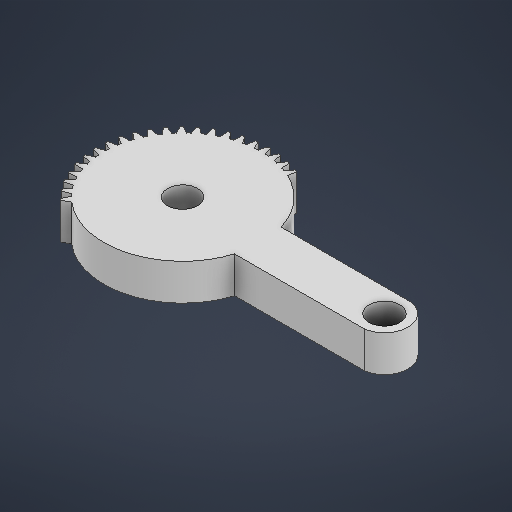
# Autodesk Inventor part: innerGear
Saved by Autodesk Inventor 2026.2 (Build 302298000, 298)
## iProperties
Created: 2026-04-07
Part Number: innerGear
Material: Generic
Document SubType Name: Modeling
Designer: Brian Wang
Density: 1 g/cm^3
Appearance: Default
Author: Brian Wang
Autodesk Inventor part; units mm, degrees
ref_plane "YZ Plane" through (0, 0, 0) normal (1, 0, 0) x (0, 1, 0)
ref_plane "XZ Plane" through (0, 0, 0) normal (0, 1, 0) x (-1, 0, 0)
ref_plane "XY Plane" through (0, 0, 0) normal (0, 0, 1) x (1, 0, 0)
sketch "Sketch1" plane through (0, 0, 0) normal (0, 1, 0) x (-1, 0, 0)
  circle A0 centre (0, 0) radius 11
  line L0 (0, 0) -> (21.5969, 0.9429) construction
  line L1 (0, 0) -> (22.384, -0.9773) construction
  line L2 (0, 0) -> (25.2479, 0) construction
  line L3 (10.9895, 0.4798) -> (12.0415, 0.1582)
  line L4 (10.9895, 0.4798) -> (12.0895, 0.4798) construction
  line L5 (10.9895, -0.4798) -> (12.0415, -0.1582)
  line L6 (12.0415, -0.1582) -> (12.0415, 0.1582)
  line L7 (10.9561, 0.9815) -> (11.9561, 1.4397)
  line L8 (11.9561, 1.4397) -> (11.9142, 1.7533)
  line L9 (10.8289, 1.9326) -> (11.9142, 1.7533)
  line L10 (10.7293, 2.4254) -> (11.6597, 3.0122)
  line L11 (11.6597, 3.0122) -> (11.5765, 3.3175)
  line L12 (10.4771, 3.3513) -> (11.5765, 3.3175)
  line L13 (10.313, 3.8266) -> (11.1574, 4.5315)
  line L14 (11.1574, 4.5315) -> (11.0345, 4.8231)
  line L15 (9.9402, 4.7109) -> (11.0345, 4.8231)
  line L16 (9.7146, 5.1602) -> (10.4581, 5.9708)
  line L17 (10.4581, 5.9708) -> (10.2976, 6.2435)
  line L18 (9.2279, 5.9872) -> (10.2976, 6.2435)
  line L19 (8.9446, 6.4026) -> (9.5741, 7.3047)
  line L20 (9.5741, 7.3047) -> (9.3789, 7.5537)
  line L21 (8.3526, 7.1578) -> (9.3789, 7.5537)
  line L22 (8.0168, 7.532) -> (8.521, 8.5096)
  line L23 (8.521, 8.5096) -> (8.2945, 8.7306)
  line L24 (7.3298, 8.2021) -> (8.2945, 8.7306)
  line L25 (6.9474, 8.5284) -> (7.3176, 9.5643)
  line L26 (7.3176, 9.5643) -> (7.0638, 9.7532)
  line L27 (6.1776, 9.1015) -> (7.0638, 9.7532)
  line L28 (5.7553, 9.3743) -> (5.9849, 10.45)
  line L29 (5.9849, 10.45) -> (5.7083, 10.6037)
  line L30 (4.9164, 9.8402) -> (5.7083, 10.6037)
  line L31 (4.4616, 10.0546) -> (4.5465, 11.1513)
  line L32 (4.5465, 11.1513) -> (4.252, 11.2669)
  line L33 (3.5683, 10.4052) -> (4.252, 11.2669)
  line L34 (3.0891, 10.5573) -> (3.0279, 11.6556)
  line L35 (3.0279, 11.6556) -> (2.7206, 11.7312)
  line L36 (2.1572, 10.7864) -> (2.7206, 11.7312)
  line L37 (1.6621, 10.8737) -> (1.4558, 11.9542)
  line L38 (1.4558, 11.9542) -> (1.1412, 11.9883)
  line L39 (0.708, 10.9772) -> (1.1412, 11.9883)
  line L40 (0.2057, 10.9981) -> (-0.142, 12.0417)
  line L41 (-0.142, 12.0417) -> (-0.4584, 12.0338)
  line L42 (-0.7536, 10.9742) -> (-0.4584, 12.0338)
  line L43 (-1.2543, 10.9283) -> (-1.7373, 11.9165)
  line L44 (-1.7373, 11.9165) -> (-2.0498, 11.8668)
  line L45 (-2.202, 10.7773) -> (-2.0498, 11.8668)
  line L46 (-2.6922, 10.6655) -> (-3.302, 11.581)
  line L47 (-3.302, 11.581) -> (-3.6051, 11.4902)
  line L48 (-3.6115, 10.3902) -> (-3.6051, 11.4902)
  line L49 (-4.0825, 10.2144) -> (-4.8083, 11.0409)
  line L50 (-4.8083, 11.0409) -> (-5.0967, 10.9108)
  line L51 (-4.9572, 9.8197) -> (-5.0967, 10.9108)
  line L52 (-5.4007, 9.5829) -> (-6.2297, 10.3059)
  line L53 (-6.2297, 10.3059) -> (-6.4983, 10.1387)
  line L54 (-6.2154, 9.0757) -> (-6.4983, 10.1387)
  line L55 (-6.6236, 8.7822) -> (-7.5411, 9.389)
  line L56 (-7.5411, 9.389) -> (-7.7852, 9.1876)
  line L57 (-7.3638, 8.1715) -> (-7.7852, 9.1876)
  line L58 (-7.7295, 7.8265) -> (-8.7194, 8.3062)
  line L59 (-8.7194, 8.3062) -> (-8.9346, 8.0743)
  line L60 (-8.3823, 7.1231) -> (-8.9346, 8.0743)
  line L61 (-8.699, 6.7326) -> (-9.7437, 7.0768)
  line L62 (-9.7437, 7.0768) -> (-9.9263, 6.8184)
  line L63 (-9.2527, 5.9488) -> (-9.9263, 6.8184)
  line L64 (-9.5148, 5.5198) -> (-10.596, 5.7225)
  line L65 (-10.596, 5.7225) -> (-10.7427, 5.4421)
  line L66 (-9.9597, 4.6695) -> (-10.7427, 5.4421)
  line L67 (-10.1627, 4.2095) -> (-11.2612, 4.2671)
  line L68 (-11.2612, 4.2671) -> (-11.3694, 3.9698)
  line L69 (-10.4909, 3.3078) -> (-11.3694, 3.9698)
  line L70 (19.4119, 54.3111) -> (-46.6371, 52.0046)
  line L71 (18.6565, 53.6502) -> (84.7457, 53.6502) construction
  line L72 (-1.8528, 64.9337) -> (-1.6772, 63.8479)
  line L73 (-1.6772, 63.8479) -> (-1.3637, 63.8049)
  line L74 (-0.9021, 64.8033) -> (-1.3637, 63.8049)
  line L75 (-0.4191, 64.7692) -> (-0.101, 63.7162)
  line L76 (-0.101, 63.7162) -> (0.2154, 63.7152)
  line L77 (0.5405, 64.766) -> (0.2154, 63.7152)
  line L78 (1.0237, 64.7963) -> (1.4786, 63.7947)
  line L79 (1.4786, 63.7947) -> (1.7924, 63.8356)
  line L80 (1.9753, 64.9203) -> (1.7924, 63.8356)
  line L81 (3.0338, 64.082) -> (3.3394, 64.1641)
  line L82 (2.4502, 65.0144) -> (3.0338, 64.082)
  line L83 (3.3769, 65.2635) -> (3.3394, 64.1641)
  line L84 (3.835, 65.4196) -> (4.5371, 64.5728)
  line L85 (4.5371, 64.5728) -> (4.8291, 64.6948)
  line L86 (4.7205, 65.7894) -> (4.8291, 64.6948)
  line L87 (5.1538, 66.0049) -> (5.962, 65.2587)
  line L88 (5.962, 65.2587) -> (6.2352, 65.4182)
  line L89 (5.9825, 66.4888) -> (6.2352, 65.4182)
  line L90 (6.3834, 66.7598) -> (7.2833, 66.1273)
  line L91 (7.2833, 66.1273) -> (7.533, 66.3217)
  line L92 (7.1406, 67.3493) -> (7.533, 66.3217)
  line L93 (7.5019, 67.671) -> (8.4778, 67.1634)
  line L94 (8.4778, 67.1634) -> (8.6995, 67.3892)
  line L95 (8.1742, 68.3557) -> (8.6995, 67.3892)
  line L96 (-3.7094, 65.4468) -> (-4.4172, 64.6047)
  line L97 (-2.3271, 65.0316) -> (-2.917, 64.1031)
  line L98 (-3.222, 64.1873) -> (-2.917, 64.1031)
  line L99 (-3.2522, 65.2869) -> (-3.222, 64.1873)
  line L100 (-3.7094, 65.4468) -> (-4.1401, 64.4346) construction
  line L101 (-4.7083, 64.7286) -> (-4.4172, 64.6047)
  line L102 (-4.5924, 65.8225) -> (-4.7083, 64.7286)
  line L103 (8.4897, 68.7224) -> (9.5243, 68.3487)
  line L104 (9.5243, 68.3487) -> (9.7141, 68.6019)
  line L105 (9.0653, 69.4902) -> (9.7141, 68.6019)
  line L106 (10.4043, 69.6622) -> (10.5589, 69.9383)
  line L107 (9.7981, 70.7328) -> (10.5589, 69.9383)
  line L108 (9.3293, 69.8954) -> (10.4043, 69.6622)
  line L109 (10.006, 71.1694) -> (11.1024, 71.0807)
  line L110 (11.1024, 71.0807) -> (11.219, 71.3749)
  line L111 (10.3596, 72.0615) -> (11.219, 71.3749)
  line L112 (10.5077, 72.5217) -> (11.6062, 72.5792)
  line L113 (11.6062, 72.5792) -> (11.6828, 72.8862)
  line L114 (10.7399, 73.4528) -> (11.6828, 72.8862)
  line L115 (10.8257, 73.9285) -> (11.9069, 74.1312)
  line L116 (11.9069, 74.1312) -> (11.9421, 74.4456)
  line L117 (10.9324, 74.8822) -> (11.9421, 74.4456)
  line L118 (10.9544, 75.365) -> (11.9992, 75.7093)
  line L119 (11.9992, 75.7093) -> (11.9924, 76.0256)
  line L120 (10.9337, 76.3244) -> (11.9924, 76.0256)
  line L121 (10.8915, 76.8058) -> (11.8814, 77.2855)
  line L122 (11.8814, 77.2855) -> (11.8327, 77.5982)
  line L123 (10.7438, 77.754) -> (11.8327, 77.5982)
  line L124 (10.6381, 78.2255) -> (11.5557, 78.8322)
  line L125 (11.5557, 78.8322) -> (11.466, 79.1357)
  line L126 (10.366, 79.1458) -> (11.466, 79.1357)
  line L127 (10.1988, 79.599) -> (11.0278, 80.322)
  line L128 (11.0278, 80.322) -> (10.8987, 80.6109)
  line L129 (9.8071, 80.475) -> (10.8987, 80.6109)
  line L130 (9.5813, 80.902) -> (10.3071, 81.7286)
  line L131 (10.3071, 81.7286) -> (10.1408, 81.9978)
  line L132 (9.0769, 81.7184) -> (10.1408, 81.9978)
  line L133 (8.7965, 82.1116) -> (9.4063, 83.0271)
  line L134 (9.4063, 83.0271) -> (9.2058, 83.2719)
  line L135 (8.1883, 82.8539) -> (9.2058, 83.2719)
  line L136 (7.8583, 83.2065) -> (8.3414, 84.1947)
  line L137 (8.3414, 84.1947) -> (8.1102, 84.4107)
  line L138 (7.1571, 83.8615) -> (8.1102, 84.4107)
  circle A1 centre (-27.7353, 75.6145) radius 2.125
  arc A2 (-28.2533, 78.823) -> (-28.265, 72.408) centre (-27.7353, 75.6145) ccw
  line L139 (-28.265, 72.408) -> (-10.2739, 72.408)
  line L140 (-28.2533, 78.823) -> (-10.2623, 78.823)
  circle A3 centre (0.1033, 75.6173) radius 2.075
  arc A4 (7.2999, 83.7372) -> (-10.2623, 78.823) centre (0.1033, 75.6173) ccw
  arc A5 (8.1883, 82.8539) -> (7.8583, 83.2065) centre (0.1033, 75.6173) ccw
  arc A6 (9.0769, 81.7184) -> (8.7965, 82.1116) centre (0.1033, 75.6173) ccw
  arc A7 (9.8071, 80.475) -> (9.5813, 80.902) centre (0.1033, 75.6173) ccw
  arc A8 (10.366, 79.1458) -> (10.1988, 79.599) centre (0.1033, 75.6173) ccw
  arc A9 (10.7438, 77.754) -> (10.6381, 78.2255) centre (0.1033, 75.6173) ccw
  arc A10 (10.9337, 76.3244) -> (10.8915, 76.8058) centre (0.1033, 75.6173) ccw
  arc A11 (10.9324, 74.8822) -> (10.9544, 75.365) centre (0.1033, 75.6173) ccw
  arc A12 (10.7399, 73.4528) -> (10.8257, 73.9285) centre (0.1033, 75.6173) ccw
  arc A13 (10.3596, 72.0615) -> (10.5077, 72.5217) centre (0.1033, 75.6173) ccw
  arc A14 (9.7981, 70.7328) -> (10.006, 71.1694) centre (0.1033, 75.6173) ccw
  arc A15 (9.0653, 69.4902) -> (9.3293, 69.8954) centre (0.1033, 75.6173) ccw
  arc A16 (8.1742, 68.3557) -> (8.4897, 68.7224) centre (0.1033, 75.6173) ccw
  arc A17 (7.1406, 67.3493) -> (7.5019, 67.671) centre (0.1033, 75.6173) ccw
  arc A18 (5.9825, 66.4888) -> (6.3834, 66.7598) centre (0.1033, 75.6173) ccw
  arc A19 (4.7205, 65.7894) -> (5.1538, 66.0049) centre (0.1033, 75.6173) ccw
  arc A20 (3.3769, 65.2635) -> (3.835, 65.4196) centre (0.1033, 75.6173) ccw
  arc A21 (1.9753, 64.9203) -> (2.4502, 65.0144) centre (0.1033, 75.6173) ccw
  arc A22 (0.5405, 64.766) -> (1.0237, 64.7963) centre (0.1033, 75.6173) ccw
  arc A23 (-0.9021, 64.8033) -> (-0.4191, 64.7692) centre (0.1033, 75.6173) ccw
  arc A24 (-2.3271, 65.0316) -> (-1.8528, 64.9337) centre (0.1033, 75.6173) ccw
  arc A25 (-10.2739, 72.408) -> (-5.0986, 66.0817) centre (0.1033, 75.6173) ccw
  arc A26 (-3.7094, 65.4468) -> (-3.2522, 65.2869) centre (0.1033, 75.6173) ccw
  arc A27 (-5.0986, 66.0817) -> (-4.7626, 65.9059) centre (0.1033, 75.6173) ccw
  arc A28 (-4.7626, 65.9059) -> (-4.5924, 65.8225) centre (0.1033, 75.6173) ccw
  point P0 (7.1571, 83.8615)
  dimension "d0" = 22
  dimension "d1" = 2.5
  dimension "d2" = 2.5
  dimension "d3" = 1.1
  dimension "d4" = 17
  dimension "d5" = 0.3164
  dimension "d8" = 160
  dimension "d15" = 4.15
  dimension "d21" = 10.85
  constraints: 282 end point, 52 point on circle, 45 point on line, 28 centre point, 3 coincident, 3 horizontal, 2 equal length, 2 symmetric about line, 1 concentric, 1 vertical, 172 other
  measures "d1" angle of L2 L0
  measures "d2" angle of L1 L2
  measures "d3" distance of L3.start L3.end
  measures "d4" angle of L3 L4
  measures "d5" distance of L5.end L6.end
  measures "d15" diameter of A3
  measures "d21" radius of A4
extrude "Extrusion1" add sketch "Sketch1" along normal blind 5 contours A24 L97 L98 L99 A26 L96 L101 L102 A28 A27 A25 L139 A2 L140 A4 L138 L137 L136 A5 L135 L134 L133 A6 L132 L131 L130 A7 L129 L128 L127 A8 L126 L125 L124 A9 L123 L122 L121 A10 L120 L119 L118 A11 L117 L116 L115 A12 L114 L113 L112 A13 L111 L110 L109 A14 L107 L106 L108 A15 L105 L104 L103 A16 L95 L94 L93 A17 L92 L91 L90 A18 L89 L88 L87 A19 L86 L85 L84 A20 L83 L81 L82 A21 L80 L79 L78 A22 L77 L76 L75 A23 L74 L73 L72
body "Solid1"
